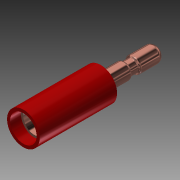
# Autodesk Inventor part: point 091 male pin red
Saved by Autodesk Inventor 2014 (Build 180170000, 170)
## iProperties
Created: 2013-07-21
Part Number: point 091 male pin red
Material: Generic
Document SubType Name: Modeling
Designer: Saville
Mass: 0.134646 g
Surface Area: 6.25479 cm^2
Volume: 0.134646 cm^3
Density: 1 g/cm^3
Appearance: Default
Author: Saville
Autodesk Inventor part; units mm, degrees
ref_plane "YZ Plane" through (0, 0, 0) normal (1, 0, 0) x (0, 1, 0)
ref_plane "XZ Plane" through (0, 0, 0) normal (0, 1, 0) x (-1, 0, 0)
ref_plane "XY Plane" through (0, 0, 0) normal (0, 0, 1) x (1, 0, 0)
sketch "Sketch1" plane through (0, 0, 0) normal (0, 0, 1) x (1, 0, 0)
  circle A0 centre (0, 0) radius 2.3813
  dimension "d0" = 4.7625
  constraints: 1 centre point, 1 coincident
  measures "d0" diameter of A0
extrude "Extrusion1" add sketch "Sketch1" along normal blind 11.2903
shell "Shell1" thickness 0.4445 removed faces 2 at (-0.7707, 0.19, 0) at (-0.7707, 0.19, 11.2903)
sketch "Sketch2" plane through (0, 0, 0) normal (0, 1, 0) x (-1, 0, 0)
  line L0 (2.3813, 11.2903) -> (2.3813, 0) projected
  line L1 (2.3813, 0) -> (1.9368, 0) projected
  line L2 (1.9368, 0) -> (1.9368, 11.2903) projected
  line L3 (1.9368, 11.2903) -> (2.3813, 11.2903) projected
  line L4 (-2.3813, 0) -> (-2.3813, 11.2903) projected
  line L5 (-2.3813, 11.2903) -> (-1.9368, 11.2903) projected
  line L6 (-1.9368, 11.2903) -> (-1.9368, 0) projected
  line L7 (-1.9368, 0) -> (-2.3813, 0) projected
  line L8 (1.9368, 0) -> (0, 0) construction
  line L9 (0, 0) -> (0, -8.1534) construction
  line L10 (1.1557, -8.1534) -> (0, -8.1534)
  line L11 (-1.1557, -8.1534) -> (-1.1557, 0) construction
  line L12 (-1.1557, 0) -> (0, 0) construction
  line L13 (-1.1557, -4.572) -> (-1.1557, -3.4925) construction
  line L14 (0.9081, -4.572) -> (0.9081, -3.4925)
  line L15 (-0.908, -4.572) -> (-0.908, -3.4925) construction
  line L16 (1.1557, -0.2302) -> (1.1557, -3.4925)
  line L17 (1.1557, -4.572) -> (1.1557, -8.1534)
  line L18 (1.1557, -4.572) -> (0.9081, -4.572)
  line L19 (0, -4.572) -> (-1.1557, -4.572) construction
  line L20 (-1.1557, -3.4925) -> (0, -3.4925) construction
  line L21 (0.9081, -3.4925) -> (1.1557, -3.4925)
  line L22 (0, -8.1534) -> (-1.1557, -8.1534) construction
  line L23 (0, 0) -> (-1.9368, 0) construction
  line L24 (0, -8.1534) -> (0, 0)
  line L25 (0, 0) -> (1.1557, 0)
  line L26 (1.1557, 0) -> (1.9368, 0)
  arc A0 (1.1557, -0.2302) -> (1.9368, 0) centre (1.1557, 1.2101) ccw
  line L27 (1.1557, -0.2302) -> (0, -0.2302) construction
  dimension "d4" = 8.1534
  dimension "d8" = 1.8161
  dimension "d13" = 1.1557
  constraints: 40 end point, 11 parallel, 9 perpendicular, 8 point on line, 5 collinear, 4 horizontal, 2 point on circle, 1 centre point, 1 tangent, 1 other
  measures "d4" distance of L8.end L9.end
  measures "d8" distance between parallel lines of L15 L14
  measures "d13" distance between parallel lines of L16 L9
revolve "Revolution1" add sketch "Sketch2" angle 360 about axis through (0, 0, 0) along (0, 0, -1) separate body contours A0 L16 L21 L14 L18 L17 L10 L24 L25 L26
fillet "Fillet1" radius 0.762 1 edges at (1.1557, 0, -8.1534)
sketch "Sketch3" plane through (0, 0, -8.1534) normal (0, 0, -1) x (-1, 0, 0)
  circle A0 centre (0, 0) radius 0.3937 projected
  circle A1 centre (0, 0) radius 0.3937 projected
  circle A2 centre (0, 0) radius 0.2586
  constraints: 1 centre point, 1 coincident
extrude "Extrusion2" cut sketch "Sketch3" against normal blind 11.2903 contours A2 bodies 1 2
fillet "Fillet2" radius 0.1016 2 edges at (0.908, 0, -4.572) (0.908, 0, -3.4925)
fillet "Fillet3" radius 0.381 2 edges at (1.1557, 0, -3.4925) (1.1557, 0, -4.572)
sketch "Sketch5" plane through (0, 0, 0) normal (0, 0, 1) x (1, 0, 0)
  circle A0 centre (0, 0) radius 0.2586 projected
  circle A1 centre (0, 0) radius 1.9368 projected
  circle A2 centre (0, 0) radius 1.6066
  dimension "d17" = 0.3302
  constraints: 1 centre point, 1 coincident
  measures "d17" radial gap between concentric circles of A1 A2
extrude "Extrusion3" add sketch "Sketch5" along normal blind 9.7028 contours A1 bodies 2
body "Solid1"
body "Solid2"
